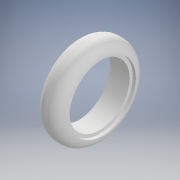
# Autodesk Inventor part: PrednjiKotač_635z_lezaj_v.2.0
Saved by Autodesk Inventor 2020 (Build 240168000, 168)
## iProperties
Created: 2020-10-01
Part Number: PrednjiKotač_635z_lezaj_v.2.0
Material: Generic
Document SubType Name: Modeling
Designer: Sičaja
Density: 1 g/cm^3
Appearance: Default
Author: Sičaja
Autodesk Inventor part; units mm, degrees
ref_plane "YZ Plane" through (0, 0, 0) normal (1, 0, 0) x (0, 1, 0)
ref_plane "XZ Plane" through (0, 0, 0) normal (0, 1, 0) x (-1, 0, 0)
ref_plane "XY Plane" through (0, 0, 0) normal (0, 0, 1) x (1, 0, 0)
sketch "Sketch1" plane through (0, 0, 0) normal (1, 0, 0) x (0, 1, 0)
  circle A0 centre (0, 0) radius 13.75
  circle A1 centre (0, 0) radius 9.5
  circle A2 centre (0, 0) radius 2.5
  circle A3 centre (0, 0) radius 10.5
  dimension "d0" = 27.5
  dimension "d1" = 19
  dimension "d2" = 5
  dimension "d3" = 21
  constraints: 4 centre point, 4 coincident
  measures "d0" diameter of A0
  measures "d1" diameter of A1
  measures "d2" diameter of A2
  measures "d3" diameter of A3
sketch "Sketch2" plane through (0, 0, 0) normal (1, 0, 0) x (0, 1, 0)
  circle A0 centre (0, 0) radius 13.75 projected
  circle A1 centre (0, 0) radius 10.5 projected
extrude "Extrusion1" add sketch "Sketch1" along normal mid plane 6 contours A3
extrude "Extrusion2" add sketch "Sketch2" along normal mid plane 8
fillet "Fillet1" radius 4 2 edges at (4, -13.75, 0) (-4, -13.75, 0)
sketch "Sketch9" plane through (3, 0, 0) normal (1, 0, 0) x (0, 0, -1)
  circle A0 centre (0, 0) radius 10.5
  circle A1 centre (0, 0) radius 8.5
  dimension "d24" = 17
  constraints: 2 centre point, 1 coincident
  measures "d24" diameter of A1
extrude "Extrusion5" add sketch "Sketch9" along normal blind 1
sketch "Sketch11" plane through (-3, 0, 0) normal (-1, 0, 0) x (0, 0, 1)
  circle A0 centre (0, 0) radius 10.7692
  circle A1 centre (0, 0) radius 10
  dimension "d30" = 20
  constraints: 2 centre point, 1 coincident
  measures "d30" diameter of A1
extrude "Extrusion7" cut sketch "Sketch11" against normal blind 2
sketch "Sketch12" plane through (-3, 0, 0) normal (-1, 0, 0) x (0, 0, 1)
  circle A0 centre (0, 0) radius 10
  circle A1 centre (0, 0) radius 10 projected
  circle A2 centre (0, 0) radius 9.25
  dimension "d33" = 18.5
  constraints: 2 centre point, 2 coincident
  measures "d33" diameter of A2
extrude "Extrusion8" add sketch "Sketch12" along normal blind 0.5
sketch "Sketch14" plane through (-3.5, 0, 0) normal (-1, 0, 0) x (0, 0, 1)
  circle A0 centre (0, 0) radius 9.25 projected
  line L0 (-9.0647, 1.8424) -> (-9.7942, 2.0184)
  circle A1 centre (0, 0) radius 10 projected
  line L1 (-9.25, 0) -> (-10, 0)
  line L2 (-9.0647, -1.8424) -> (-9.7942, -2.0184)
  constraints: 6 end point, 4 point on circle, 2 symmetric about line, 1 horizontal
extrude "Extrusion9" cut sketch "Sketch14" against normal blind 2 contours A0 L1 A1 L0 | L2 A1 L1 A0
pattern_circular "Circular Pattern2" count 10 over 360 about axis through (-3.5, 0, 0) along (1, 0, 0) of "Extrusion9"
chamfer "Chamfer2" distance 0.22 distance2 0.4 1 edges at (-3.5, 2.8584, -8.7973) measured on face at (-3.5, 3.1219, -9.2303)
chamfer "Chamfer3" distance 0.22 distance2 0.4 1 edges at (-3.5, -2.8584, -8.7973) measured on face at (-3.5, -3.1219, -9.2303)
chamfer "Chamfer4" distance 0.22 distance2 0.4 1 edges at (-3.5, -7.4834, -5.437) measured on face at (-3.5, -7.9511, -5.6325)
chamfer "Chamfer5" distance 0.22 distance2 0.4 1 edges at (-3.5, -9.25, 0) measured on face at (-3.5, -9.7432, 0.1168)
chamfer "Chamfer6" distance 0.22 distance2 0.4 1 edges at (-3.5, -7.4834, 5.437) measured on face at (-3.5, -7.9511, 5.6325)
chamfer "Chamfer7" distance 0.22 distance2 0.4 1 edges at (-3.5, -2.8584, 8.7973) measured on face at (-3.5, -3.1219, 9.2303)
chamfer "Chamfer8" distance 0.22 distance2 0.4 1 edges at (-3.5, 2.8584, 8.7973) measured on face at (-3.5, 3.1219, 9.2303)
chamfer "Chamfer9" distance 0.22 distance2 0.4 1 edges at (-3.5, 7.4834, 5.437) measured on face at (-3.5, 7.9511, 5.6325)
chamfer "Chamfer10" distance 0.22 distance2 0.4 1 edges at (-3.5, 9.25, 0) measured on face at (-3.5, 9.7432, -0.1168)
chamfer "Chamfer11" distance 0.22 distance2 0.4 1 edges at (-3.5, 7.4834, -5.437) measured on face at (-3.5, 7.9511, -5.6325)
body "Solid1"
